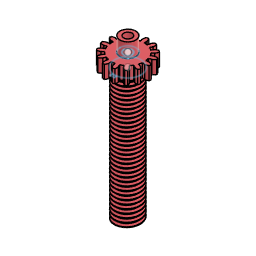
종속기어 (Autodesk Fusion 360 design; units mm, degrees)
Autodesk Fusion 360 part; units mm, degrees
sketch "스케치1" plane through (0, 0, 0) normal (0, 0, 1) x (1, 0, 0)
  spline S0 degree 5 poles (7.217568, -0.799079) (7.217624, -0.799084) (7.217742, -0.799096) (7.21794, -0.799116) (7.218244, -0.799144) (7.218692, -0.799184) (7.219206, -0.799229) (7.219786, -0.799277) (7.220433, -0.79933) (7.221146, -0.799386) (7.221923, -0.799444) (7.222764, -0.799505) (7.223669, -0.799567) (7.224637, -0.799631) (7.225668, -0.799696) (7.226762, -0.799762) (7.227917, -0.799827) (7.229133, -0.799893) (7.230411, -0.799958) (7.231749, -0.800023) (7.233147, -0.800086) (7.234604, -0.800147) (7.236121, -0.800206) (7.237696, -0.800263) (7.239329, -0.800318) (7.24102, -0.800369) (7.242769, -0.800417) (7.244574, -0.800461) (7.246436, -0.800501) (7.248354, -0.800537) (7.250328, -0.800569) (7.252358, -0.800595) (7.254442, -0.800616) (7.256581, -0.800632) (7.258774, -0.800641) (7.26102, -0.800645) (7.26332, -0.800642) (7.265674, -0.800632) (7.26808, -0.800615) (7.270538, -0.800591) (7.273048, -0.800559) (7.27561, -0.80052) (7.278223, -0.800472) (7.280887, -0.800416) (7.283601, -0.800352) (7.286366, -0.800278) (7.28918, -0.800195) (7.292044, -0.800103) (7.294957, -0.800002) (7.297919, -0.79989) (7.30093, -0.799768) (7.303989, -0.799636) (7.307095, -0.799493) (7.310249, -0.799339) (7.313451, -0.799175) (7.316699, -0.798999) (7.319994, -0.798811) (7.323336, -0.798612) (7.326723, -0.798401) (7.330156, -0.798177) (7.333634, -0.797941) (7.337158, -0.797693) (7.340726, -0.797432) (7.344339, -0.797157) (7.347996, -0.79687) (7.351697, -0.796569) (7.355442, -0.796254) (7.35923, -0.795926) (7.363061, -0.795584) (7.366935, -0.795227) (7.370851, -0.794856) (7.37481, -0.794471) (7.378811, -0.794071) (7.382853, -0.793656) (7.386937, -0.793225) (7.391062, -0.79278) (7.395228, -0.792319) (7.399434, -0.791842) (7.403681, -0.79135) (7.407968, -0.790841) (7.412295, -0.790317) (7.416662, -0.789776) (7.421067, -0.789219) (7.425512, -0.788645) (7.429996, -0.788054) (7.434519, -0.787446) (7.439079, -0.786821) (7.443678, -0.786179) (7.448315, -0.785519) (7.452989, -0.784842) (7.457701, -0.784147) (7.46245, -0.783435) (7.467236, -0.782704) (7.472058, -0.781955) (7.476917, -0.781188) (7.481812, -0.780402) (7.486743, -0.779598) (7.49171, -0.778775) (7.496712, -0.777933) (7.501749, -0.777072) (7.506822, -0.776192) (7.511929, -0.775293) (7.517071, -0.774375) (7.522248, -0.773436) (7.527458, -0.772479) (7.532703, -0.771501) (7.537981, -0.770504) (7.543292, -0.769486) (7.548637, -0.768449) (7.554015, -0.767391) (7.559426, -0.766312) (7.56487, -0.765214) (7.570345, -0.764094) (7.575854, -0.762954) (7.581394, -0.761793) (7.586966, -0.760611) (7.592569, -0.759408) (7.598204, -0.758183) (7.60387, -0.756938) (7.609567, -0.755671) (7.615295, -0.754382) (7.621053, -0.753072) (7.626842, -0.75174) (7.632661, -0.750387) (7.63851, -0.749011) (7.644389, -0.747613) (7.650297, -0.746193) (7.656234, -0.744751) (7.662201, -0.743287) (7.668197, -0.7418) (7.674222, -0.74029) (7.680275, -0.738758) (7.686357, -0.737204) (7.692466, -0.735626) (7.698604, -0.734025) (7.70477, -0.732402) (7.710964, -0.730755) (7.717184, -0.729085) (7.723433, -0.727392) (7.729708, -0.725676) (7.73601, -0.723936) (7.742339, -0.722173) (7.748695, -0.720385) (7.755076, -0.718575) (7.761484, -0.71674) (7.767919, -0.714882) (7.774378, -0.712999) (7.780864, -0.711093) (7.787375, -0.709162) (7.793911, -0.707208) (7.800473, -0.705229) (7.807059, -0.703225) (7.81367, -0.701198) (7.820306, -0.699145) (7.826966, -0.697068) (7.833651, -0.694967) (7.840359, -0.692841) (7.847092, -0.69069) (7.853848, -0.688514) (7.860628, -0.686313) (7.867431, -0.684087) (7.874257, -0.681837) (7.881107, -0.679561) (7.887979, -0.677259) (7.894874, -0.674933) (7.901792, -0.672581) (7.908732, -0.670204) (7.915694, -0.667801) (7.922679, -0.665373) (7.929685, -0.662919) (7.936713, -0.660439) (7.943763, -0.657934) (7.950834, -0.655403) (7.957926, -0.652846) (7.965039, -0.650264) (7.972174, -0.647655) (7.979329, -0.64502) (7.986505, -0.642359) (7.993701, -0.639672) (8.000917, -0.636959) (8.008154, -0.63422) (8.015411, -0.631454) (8.022688, -0.628662) (8.029984, -0.625843) (8.0373, -0.622999) (8.044635, -0.620127) (8.051989, -0.617229) (8.059363, -0.614304) (8.066755, -0.611353) (8.074167, -0.608375) (8.081596, -0.60537) (8.089045, -0.602339) (8.096511, -0.59928) (8.103996, -0.596195) (8.111499, -0.593082) (8.11902, -0.589943) (8.126558, -0.586776) (8.134115, -0.583583) (8.141688, -0.580362) (8.149279, -0.577114) (8.156887, -0.573839) (8.164512, -0.570537) (8.172154, -0.567207) (8.179812, -0.56385) (8.187487, -0.560465) (8.195179, -0.557053) (8.202887, -0.553614) (8.210611, -0.550147) (8.218351, -0.546652) (8.226106, -0.54313) (8.233878, -0.539581) (8.241665, -0.536003) (8.249468, -0.532398) (8.257285, -0.528765) (8.265118, -0.525104) (8.272966, -0.521416) (8.280829, -0.517699) (8.288707, -0.513955) (8.296599, -0.510183) (8.304506, -0.506382) (8.312427, -0.502554) (8.320362, -0.498698) (8.328312, -0.494814) (8.336275, -0.490901) (8.344252, -0.486961) (8.352243, -0.482992) (8.360247, -0.478995) (8.368265, -0.47497) (8.376295, -0.470916) (8.384339, -0.466835) (8.392396, -0.462725) (8.400466, -0.458587) (8.408549, -0.45442) (8.416644, -0.450225) (8.424752, -0.446001) (8.432872, -0.441749) (8.441004, -0.437469) (8.449148, -0.43316) (8.457304, -0.428822) (8.465472, -0.424456) (8.473651, -0.420062) (8.480205, -0.416523) (8.485125, -0.413856) (8.488407, -0.412073) (8.490049, -0.41118) knots 0 0 0 0 0 0 0.00416667 0.00833333 0.0125 0.01666667 0.02083333 0.025 0.02916667 0.03333333 0.0375 0.04166667 0.04583333 0.05 0.05416667 0.05833333 0.0625 0.06666667 0.07083333 0.075 0.07916667 0.08333333 0.0875 0.09166667 0.09583333 0.1 0.10416667 0.10833333 0.1125 0.11666667 0.12083333 0.125 0.12916667 0.13333333 0.1375 0.14166667 0.14583333 0.15 0.15416667 0.15833333 0.1625 0.16666667 0.17083333 0.175 0.17916667 0.18333333 0.1875 0.19166667 0.19583333 0.2 0.20416667 0.20833333 0.2125 0.21666667 0.22083333 0.225 0.22916667 0.23333333 0.2375 0.24166667 0.24583333 0.25 0.25416667 0.25833333 0.2625 0.26666667 0.27083333 0.275 0.27916667 0.28333333 0.2875 0.29166667 0.29583333 0.3 0.30416667 0.30833333 0.3125 0.31666667 0.32083333 0.325 0.32916667 0.33333333 0.3375 0.34166667 0.34583333 0.35 0.35416667 0.35833333 0.3625 0.36666667 0.37083333 0.375 0.37916667 0.38333333 0.3875 0.39166667 0.39583333 0.4 0.40416667 0.40833333 0.4125 0.41666667 0.42083333 0.425 0.42916667 0.43333333 0.4375 0.44166667 0.44583333 0.45 0.45416667 0.45833333 0.4625 0.46666667 0.47083333 0.475 0.47916667 0.48333333 0.4875 0.49166667 0.49583333 0.5 0.50416667 0.50833333 0.5125 0.51666667 0.52083333 0.525 0.52916667 0.53333333 0.5375 0.54166667 0.54583333 0.55 0.55416667 0.55833333 0.5625 0.56666667 0.57083333 0.575 0.57916667 0.58333333 0.5875 0.59166667 0.59583333 0.6 0.60416667 0.60833333 0.6125 0.61666667 0.62083333 0.625 0.62916667 0.63333333 0.6375 0.64166667 0.64583333 0.65 0.65416667 0.65833333 0.6625 0.66666667 0.67083333 0.675 0.67916667 0.68333333 0.6875 0.69166667 0.69583333 0.7 0.70416667 0.70833333 0.7125 0.71666667 0.72083333 0.725 0.72916667 0.73333333 0.7375 0.74166667 0.74583333 0.75 0.75416667 0.75833333 0.7625 0.76666667 0.77083333 0.775 0.77916667 0.78333333 0.7875 0.79166667 0.79583333 0.8 0.80416667 0.80833333 0.8125 0.81666667 0.82083333 0.825 0.82916667 0.83333333 0.8375 0.84166667 0.84583333 0.85 0.85416667 0.85833333 0.8625 0.86666667 0.87083333 0.875 0.87916667 0.88333333 0.8875 0.89166667 0.89583333 0.9 0.90416667 0.90833333 0.9125 0.91666667 0.92083333 0.925 0.92916667 0.93333333 0.9375 0.94166667 0.94583333 0.95 0.95416667 0.95833333 0.9625 0.96666667 0.97083333 0.975 0.97916667 0.98333333 0.9875 0.99166667 0.99583333 1 1 1 1 1 1
  spline S1 degree 5 poles (7.217568, 0.799079) (7.217624, 0.799084) (7.217742, 0.799096) (7.21794, 0.799116) (7.218244, 0.799144) (7.218692, 0.799184) (7.219206, 0.799229) (7.219786, 0.799277) (7.220433, 0.79933) (7.221146, 0.799386) (7.221923, 0.799444) (7.222764, 0.799505) (7.223669, 0.799567) (7.224637, 0.799631) (7.225668, 0.799696) (7.226762, 0.799762) (7.227917, 0.799827) (7.229133, 0.799893) (7.230411, 0.799958) (7.231749, 0.800023) (7.233147, 0.800086) (7.234604, 0.800147) (7.236121, 0.800206) (7.237696, 0.800263) (7.239329, 0.800318) (7.24102, 0.800369) (7.242769, 0.800417) (7.244574, 0.800461) (7.246436, 0.800501) (7.248354, 0.800537) (7.250328, 0.800569) (7.252358, 0.800595) (7.254442, 0.800616) (7.256581, 0.800632) (7.258774, 0.800641) (7.26102, 0.800645) (7.26332, 0.800642) (7.265674, 0.800632) (7.26808, 0.800615) (7.270538, 0.800591) (7.273048, 0.800559) (7.27561, 0.80052) (7.278223, 0.800472) (7.280887, 0.800416) (7.283601, 0.800352) (7.286366, 0.800278) (7.28918, 0.800195) (7.292044, 0.800103) (7.294957, 0.800002) (7.297919, 0.79989) (7.30093, 0.799768) (7.303989, 0.799636) (7.307095, 0.799493) (7.310249, 0.799339) (7.313451, 0.799175) (7.316699, 0.798999) (7.319994, 0.798811) (7.323336, 0.798612) (7.326723, 0.798401) (7.330156, 0.798177) (7.333634, 0.797941) (7.337158, 0.797693) (7.340726, 0.797432) (7.344339, 0.797157) (7.347996, 0.79687) (7.351697, 0.796569) (7.355442, 0.796254) (7.35923, 0.795926) (7.363061, 0.795584) (7.366935, 0.795227) (7.370851, 0.794856) (7.37481, 0.794471) (7.378811, 0.794071) (7.382853, 0.793656) (7.386937, 0.793225) (7.391062, 0.79278) (7.395228, 0.792319) (7.399434, 0.791842) (7.403681, 0.79135) (7.407968, 0.790841) (7.412295, 0.790317) (7.416662, 0.789776) (7.421067, 0.789219) (7.425512, 0.788645) (7.429996, 0.788054) (7.434519, 0.787446) (7.439079, 0.786821) (7.443678, 0.786179) (7.448315, 0.785519) (7.452989, 0.784842) (7.457701, 0.784147) (7.46245, 0.783435) (7.467236, 0.782704) (7.472058, 0.781955) (7.476917, 0.781188) (7.481812, 0.780402) (7.486743, 0.779598) (7.49171, 0.778775) (7.496712, 0.777933) (7.501749, 0.777072) (7.506822, 0.776192) (7.511929, 0.775293) (7.517071, 0.774375) (7.522248, 0.773436) (7.527458, 0.772479) (7.532703, 0.771501) (7.537981, 0.770504) (7.543292, 0.769486) (7.548637, 0.768449) (7.554015, 0.767391) (7.559426, 0.766312) (7.56487, 0.765214) (7.570345, 0.764094) (7.575854, 0.762954) (7.581394, 0.761793) (7.586966, 0.760611) (7.592569, 0.759408) (7.598204, 0.758183) (7.60387, 0.756938) (7.609567, 0.755671) (7.615295, 0.754382) (7.621053, 0.753072) (7.626842, 0.75174) (7.632661, 0.750387) (7.63851, 0.749011) (7.644389, 0.747613) (7.650297, 0.746193) (7.656234, 0.744751) (7.662201, 0.743287) (7.668197, 0.7418) (7.674222, 0.74029) (7.680275, 0.738758) (7.686357, 0.737204) (7.692466, 0.735626) (7.698604, 0.734025) (7.70477, 0.732402) (7.710964, 0.730755) (7.717184, 0.729085) (7.723433, 0.727392) (7.729708, 0.725676) (7.73601, 0.723936) (7.742339, 0.722173) (7.748695, 0.720385) (7.755076, 0.718575) (7.761484, 0.71674) (7.767919, 0.714882) (7.774378, 0.712999) (7.780864, 0.711093) (7.787375, 0.709162) (7.793911, 0.707208) (7.800473, 0.705229) (7.807059, 0.703225) (7.81367, 0.701198) (7.820306, 0.699145) (7.826966, 0.697068) (7.833651, 0.694967) (7.840359, 0.692841) (7.847092, 0.69069) (7.853848, 0.688514) (7.860628, 0.686313) (7.867431, 0.684087) (7.874257, 0.681837) (7.881107, 0.679561) (7.887979, 0.677259) (7.894874, 0.674933) (7.901792, 0.672581) (7.908732, 0.670204) (7.915694, 0.667801) (7.922679, 0.665373) (7.929685, 0.662919) (7.936713, 0.660439) (7.943763, 0.657934) (7.950834, 0.655403) (7.957926, 0.652846) (7.965039, 0.650264) (7.972174, 0.647655) (7.979329, 0.64502) (7.986505, 0.642359) (7.993701, 0.639672) (8.000917, 0.636959) (8.008154, 0.63422) (8.015411, 0.631454) (8.022688, 0.628662) (8.029984, 0.625843) (8.0373, 0.622999) (8.044635, 0.620127) (8.051989, 0.617229) (8.059363, 0.614304) (8.066755, 0.611353) (8.074167, 0.608375) (8.081596, 0.60537) (8.089045, 0.602339) (8.096511, 0.59928) (8.103996, 0.596195) (8.111499, 0.593082) (8.11902, 0.589943) (8.126558, 0.586776) (8.134115, 0.583583) (8.141688, 0.580362) (8.149279, 0.577114) (8.156887, 0.573839) (8.164512, 0.570537) (8.172154, 0.567207) (8.179812, 0.56385) (8.187487, 0.560465) (8.195179, 0.557053) (8.202887, 0.553614) (8.210611, 0.550147) (8.218351, 0.546652) (8.226106, 0.54313) (8.233878, 0.539581) (8.241665, 0.536003) (8.249468, 0.532398) (8.257285, 0.528765) (8.265118, 0.525104) (8.272966, 0.521416) (8.280829, 0.517699) (8.288707, 0.513955) (8.296599, 0.510183) (8.304506, 0.506382) (8.312427, 0.502554) (8.320362, 0.498698) (8.328312, 0.494814) (8.336275, 0.490901) (8.344252, 0.486961) (8.352243, 0.482992) (8.360247, 0.478995) (8.368265, 0.47497) (8.376295, 0.470916) (8.384339, 0.466835) (8.392396, 0.462725) (8.400466, 0.458587) (8.408549, 0.45442) (8.416644, 0.450225) (8.424752, 0.446001) (8.432872, 0.441749) (8.441004, 0.437469) (8.449148, 0.43316) (8.457304, 0.428822) (8.465472, 0.424456) (8.473651, 0.420062) (8.480205, 0.416523) (8.485125, 0.413856) (8.488407, 0.412073) (8.490049, 0.41118) knots 0 0 0 0 0 0 0.00416667 0.00833333 0.0125 0.01666667 0.02083333 0.025 0.02916667 0.03333333 0.0375 0.04166667 0.04583333 0.05 0.05416667 0.05833333 0.0625 0.06666667 0.07083333 0.075 0.07916667 0.08333333 0.0875 0.09166667 0.09583333 0.1 0.10416667 0.10833333 0.1125 0.11666667 0.12083333 0.125 0.12916667 0.13333333 0.1375 0.14166667 0.14583333 0.15 0.15416667 0.15833333 0.1625 0.16666667 0.17083333 0.175 0.17916667 0.18333333 0.1875 0.19166667 0.19583333 0.2 0.20416667 0.20833333 0.2125 0.21666667 0.22083333 0.225 0.22916667 0.23333333 0.2375 0.24166667 0.24583333 0.25 0.25416667 0.25833333 0.2625 0.26666667 0.27083333 0.275 0.27916667 0.28333333 0.2875 0.29166667 0.29583333 0.3 0.30416667 0.30833333 0.3125 0.31666667 0.32083333 0.325 0.32916667 0.33333333 0.3375 0.34166667 0.34583333 0.35 0.35416667 0.35833333 0.3625 0.36666667 0.37083333 0.375 0.37916667 0.38333333 0.3875 0.39166667 0.39583333 0.4 0.40416667 0.40833333 0.4125 0.41666667 0.42083333 0.425 0.42916667 0.43333333 0.4375 0.44166667 0.44583333 0.45 0.45416667 0.45833333 0.4625 0.46666667 0.47083333 0.475 0.47916667 0.48333333 0.4875 0.49166667 0.49583333 0.5 0.50416667 0.50833333 0.5125 0.51666667 0.52083333 0.525 0.52916667 0.53333333 0.5375 0.54166667 0.54583333 0.55 0.55416667 0.55833333 0.5625 0.56666667 0.57083333 0.575 0.57916667 0.58333333 0.5875 0.59166667 0.59583333 0.6 0.60416667 0.60833333 0.6125 0.61666667 0.62083333 0.625 0.62916667 0.63333333 0.6375 0.64166667 0.64583333 0.65 0.65416667 0.65833333 0.6625 0.66666667 0.67083333 0.675 0.67916667 0.68333333 0.6875 0.69166667 0.69583333 0.7 0.70416667 0.70833333 0.7125 0.71666667 0.72083333 0.725 0.72916667 0.73333333 0.7375 0.74166667 0.74583333 0.75 0.75416667 0.75833333 0.7625 0.76666667 0.77083333 0.775 0.77916667 0.78333333 0.7875 0.79166667 0.79583333 0.8 0.80416667 0.80833333 0.8125 0.81666667 0.82083333 0.825 0.82916667 0.83333333 0.8375 0.84166667 0.84583333 0.85 0.85416667 0.85833333 0.8625 0.86666667 0.87083333 0.875 0.87916667 0.88333333 0.8875 0.89166667 0.89583333 0.9 0.90416667 0.90833333 0.9125 0.91666667 0.92083333 0.925 0.92916667 0.93333333 0.9375 0.94166667 0.94583333 0.95 0.95416667 0.95833333 0.9625 0.96666667 0.97083333 0.975 0.97916667 0.98333333 0.9875 0.99166667 0.99583333 1 1 1 1 1 1
  spline S2 degree 5 poles (7.217011, -0.799022) (7.217033, -0.799024) (7.217078, -0.799028) (7.217144, -0.799035) (7.217234, -0.799044) (7.217345, -0.799056) (7.217434, -0.799065) (7.217501, -0.799072) (7.217546, -0.799076) (7.217568, -0.799079) knots 0 0 0 0 0 0 0.2 0.4 0.6 0.8 1 1 1 1 1 1
  spline S3 degree 5 poles (7.217011, 0.799022) (7.217033, 0.799024) (7.217078, 0.799028) (7.217144, 0.799035) (7.217234, 0.799044) (7.217345, 0.799056) (7.217434, 0.799065) (7.217501, 0.799072) (7.217546, 0.799076) (7.217568, 0.799079) knots 0 0 0 0 0 0 0.2 0.4 0.6 0.8 1 1 1 1 1 1
  line L0 (0, 0) -> (7.217011, -0.799022)
  line L1 (0, 0) -> (7.217011, 0.799022)
  arc A0 (8.490049, -0.41118) -> (8.490049, 0.41118) centre (0, 0) ccw
  point P0 (7.219241, -0.799231)
  point P1 (7.222032, -0.799452)
  point P2 (7.225944, -0.799712)
  point P3 (7.230976, -0.799985)
  point P4 (7.237131, -0.800242)
  point P5 (7.244408, -0.800456)
  point P6 (7.252807, -0.800599)
  point P7 (7.262327, -0.800642)
  point P8 (7.272967, -0.800559)
  point P9 (7.284724, -0.800321)
  point P10 (7.297598, -0.7999)
  point P11 (7.311583, -0.79927)
  point P12 (7.326679, -0.798401)
  point P13 (7.342879, -0.797267)
  point P14 (7.360181, -0.79584)
  point P15 (7.378578, -0.794092)
  point P16 (7.398066, -0.791996)
  point P17 (7.418638, -0.789524)
  point P18 (7.440288, -0.786651)
  point P19 (7.46301, -0.783347)
  point P20 (7.486795, -0.779586)
  point P21 (7.511635, -0.775342)
  point P22 (7.537522, -0.770587)
  point P23 (7.564447, -0.765296)
  point P24 (7.592401, -0.75944)
  point P25 (7.621373, -0.752995)
  point P26 (7.651353, -0.745934)
  point P27 (7.68233, -0.738231)
  point P28 (7.714292, -0.72986)
  point P29 (7.747228, -0.720795)
  point P30 (7.781125, -0.711012)
  point P31 (7.815969, -0.700484)
  point P32 (7.851749, -0.689187)
  point P33 (7.888449, -0.677097)
  point P34 (7.926055, -0.664188)
  point P35 (7.964553, -0.650436)
  point P36 (8.003928, -0.635817)
  point P37 (8.044162, -0.620308)
  point P38 (8.085241, -0.603884)
  point P39 (8.127148, -0.586523)
  point P40 (8.169865, -0.568201)
  point P41 (8.213375, -0.548896)
  point P42 (8.25766, -0.528585)
  point P43 (8.302701, -0.507246)
  point P44 (8.348481, -0.484858)
  point P45 (8.394978, -0.461398)
  point P46 (8.442174, -0.436845)
  point P47 (7.219241, 0.799231)
  point P48 (7.222032, 0.799452)
  point P49 (7.225944, 0.799712)
  point P50 (7.230976, 0.799985)
  point P51 (7.237131, 0.800242)
  point P52 (7.244408, 0.800456)
  point P53 (7.252807, 0.800599)
  point P54 (7.262327, 0.800642)
  point P55 (7.272967, 0.800559)
  point P56 (7.284724, 0.800321)
  point P57 (7.297598, 0.7999)
  point P58 (7.311583, 0.79927)
  point P59 (7.326679, 0.798401)
  point P60 (7.342879, 0.797267)
  point P61 (7.360181, 0.79584)
  point P62 (7.378578, 0.794092)
  point P63 (7.398066, 0.791996)
  point P64 (7.418638, 0.789524)
  point P65 (7.440288, 0.786651)
  point P66 (7.46301, 0.783347)
  point P67 (7.486795, 0.779586)
  point P68 (7.511635, 0.775342)
  point P69 (7.537522, 0.770587)
  point P70 (7.564447, 0.765296)
  point P71 (7.592401, 0.75944)
  point P72 (7.621373, 0.752995)
  point P73 (7.651353, 0.745934)
  point P74 (7.68233, 0.738231)
  point P75 (7.714292, 0.72986)
  point P76 (7.747228, 0.720795)
  point P77 (7.781125, 0.711012)
  point P78 (7.815969, 0.700484)
  point P79 (7.851749, 0.689187)
  point P80 (7.888449, 0.677097)
  point P81 (7.926055, 0.664188)
  point P82 (7.964553, 0.650436)
  point P83 (8.003928, 0.635817)
  point P84 (8.044162, 0.620308)
  point P85 (8.085241, 0.603884)
  point P86 (8.127148, 0.586523)
  point P87 (8.169865, 0.568201)
  point P88 (8.213375, 0.548896)
  point P89 (8.25766, 0.528585)
  point P90 (8.302701, 0.507246)
  point P91 (8.348481, 0.484858)
  point P92 (8.394978, 0.461398)
  point P93 (8.442174, 0.436845)
sketch "스케치2" plane through (0, 0, 0) normal (0, 0, 1) x (1, 0, 0)
  circle A0 centre (0, 0) radius 6.25
extrude "돌출1" add sketch "스케치2" along normal blind 5 contours A0 picked at (0.027358, -1.484088) makes body 1
extrude "돌출2" add sketch "스케치1" along normal blind 5 separate body contours S0 S1 L0 L1 A0 picked at (4.811712, 0) makes body 2
pattern_circular "C-패턴1" count 15 over 360 about axis through (0, 0, 1.75) along (0, 0, 1) of "돌출2" makes body 3 at (2.306197, 0.735218, 1.666667) makes body 4 at (1.807776, 1.60967, 1.666667) makes body 5 at (1.993547, 4.411591, 3.333333) makes body 6 at (0.01342, 2.420519, 1.666667) makes body 7 at (-0.972254, 2.216712, 1.666667) makes body 8 at (-1.789816, 1.629616, 1.666667) makes body 9 at (-2.297903, 0.760745, 1.666667) makes body 10 at (-2.408661, -0.239667, 1.666667) makes body 11 at (-2.102941, -1.198637, 1.666667) makes body 12 at (-1.433602, -1.950353, 1.666667) makes body 13 at (-0.516381, -2.364834, 1.666667) makes body 14 at (0.490127, -2.370415, 1.666667) makes body 15 at (1.411888, -1.966129, 1.666667) makes body 16 at (2.089521, -1.221881, 1.666667)
combine "결합1" operation add target body 1 tool bodies 2 3 4 5 6 7 8 9 10 11 12 13 14 15 16
sketch "스케치3" plane through (0, 0, 0) normal (0, 0, 1) x (1, 0, 0)
  line L0 (0, 0) -> (49.936528, 0) construction
  line L1 (49.936528, 0) -> (49.936528, 3) construction
  line L2 (49.936528, 3) -> (0, 3) construction
  line L3 (0, 3) -> (0, 0) construction
  constraint perpendicular L0 L1
  constraint parallel L0 L2
  constraint parallel L1 L3
sketch "sketch 1333" plane through (0, 0, 5) normal (0, 0, 1) x (-1, 0, 0)
  circle A0 centre (0, 0) radius 1.6
extrude "돌출3" cut sketch "sketch 1333" against normal blind 5 contours A0 picked at (1.190961, -0.099121) bodies 1
sketch "sketch 1346" plane through (0, 0, 5) normal (0, 0, 1) x (-1, 0, 0)
  circle A0 centre (0, 0) radius 1.6
  circle A1 centre (0, 0) radius 3
extrude "돌출4" add sketch "sketch 1346" along normal blind 5.5 contours A1 picked at (2.516207, -0.228531) bodies 1
sketch "sketch 1361" plane through (0.324673, 5.991209, 0) normal (0, 0, -1) x (0.99853487, -0.05411211, 0)
  circle A0 centre (0, 6) radius 5
extrude "돌출5" add sketch "sketch 1361" along normal blind 50 contours A0 picked at (-0.165052, 7.121549) bodies 1
thread "나사산1" "ISO Metric profile 10.0 M10x1.5 6g" major diameter 9.85 minor diameter 8.141 pitch 1.5 angle 60 modelled right hand crest width 0.217683 on face at (4.994804, 0.227894, -16.666667) crest through (4.917784, -0.266502, 0.375) on bodies 1
sketch "sketch 1373" plane through (-0.023428, 5.999955, 0) normal (0, 0, -1) x (0.99999238, 0.00390467, 0)
  line L0 (-0.760039, 11.955992) -> (0.760039, 11.955992)
  line L1 (-0.760039, 11.254417) -> (-0.760039, 11.955992)
  line L2 (0.760039, 11.254417) -> (-0.760039, 11.254417)
  line L3 (0.760039, 11.955992) -> (0.760039, 11.254417)
extrude "돌출6" add sketch "sketch 1373" along normal blind 1 contours L0 L1 L2 L3 picked at (-0.253346, 11.722134) bodies 1
